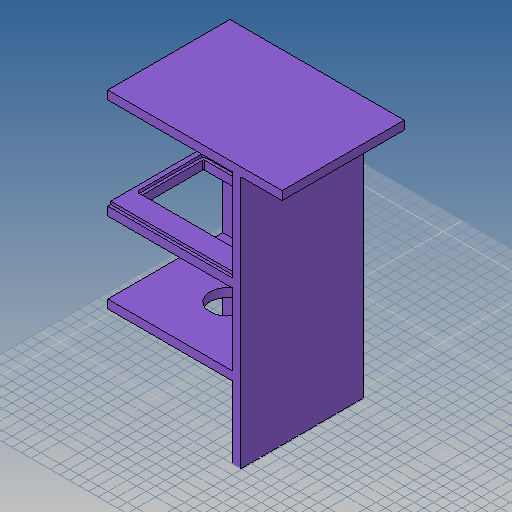
# Autodesk Inventor part: Korpus_Einbau
Saved by Autodesk Inventor 2019 (Build 230136000, 136)
## iProperties
Created: 2020-08-02
Part Number: Korpus_Einbau
Material: Generisch
Document SubType Name: Modeling
Designer: Stefan
Density: 1 g/cm^3
Appearance: Violett
Mass: 7933.41 g
Surface Area: 9734.6 cm^2
Volume: 7933.41 cm^3
Author: Stefan
Autodesk Inventor part; units mm, degrees
ref_plane "YZ Plane" through (0, 0, 0) normal (1, 0, 0) x (0, 1, 0)
ref_plane "XZ Plane" through (0, 0, 0) normal (0, 1, 0) x (-1, 0, 0)
ref_plane "XY Plane" through (0, 0, 0) normal (0, 0, 1) x (1, 0, 0)
sketch "Skizze1" plane through (0, 0, 0) normal (1, 0, 0) x (0, 1, 0)
  line L0 (0, 0) -> (18, 0)
  line L1 (18, 0) -> (18, 240)
  line L2 (18, 240) -> (0, 240)
  line L3 (0, 240) -> (0, 0)
  line L4 (378, 0) -> (-150, 0)
  line L5 (-150, -15) -> (378, -15)
  line L6 (378, -15) -> (378, 0)
  line L7 (378, -15) -> (378, 240)
  line L8 (378, 240) -> (396, 240)
  line L9 (396, 240) -> (396, -15)
  line L10 (396, -15) -> (378, -15)
  line L11 (-150, 0) -> (-150, -15)
  line L12 (186, 0) -> (168, 0)
  line L13 (168, 0) -> (168, 240)
  line L14 (168, 240) -> (186, 240)
  line L15 (186, 240) -> (186, 0)
  dimension "d0" = 18
  dimension "d1" = 15
  dimension "d2" = 18
  dimension "d5" = 255
  dimension "d6" = 360
  dimension "d23" = 150
  dimension "d49" = 18
  dimension "d50" = 150
  dimension "d51" = 192
  dimension "d52" = 255
  constraints: 32 end point, 6 parallel, 4 horizontal, 3 collinear, 2 perpendicular, 2 point on line, 1 vertical
  measures "d0" distance between parallel lines of L3 L1
  measures "d1" distance of L5.end L4.start
  measures "d2" distance of L7.end L8.end
  measures "d5" distance between parallel lines of L5 L2
  measures "d6" distance between parallel lines of L1 L7
  measures "d23" distance between parallel lines of L11 L3
  measures "d49" distance between parallel lines of L13 L15
  measures "d50" distance between parallel lines of L1 L13
  measures "d51" distance between parallel lines of L15 L7
  measures "d52" distance between parallel lines of L14 L5
extrude "Extrusion1" add sketch "Skizze1" against normal blind 260
extrude "Extrusion7" add sketch "Skizze1" along normal blind 104 contours L6 L7 L8 L9 L10
sketch "Skizze2" plane through (0, 0, 0) normal (0, -1, 0) x (1, 0, 0)
  line L0 (0, 0) -> (-260, 0) projected
  line L1 (0, 240) -> (-260, 240) projected
  circle A0 centre (-130, 120) radius 36.5
  line L2 (-130, 240) -> (-130, 0) construction
  point P0 (240, 0)
  dimension "d9" = 73
  constraints: 3 midpoint, 2 end point, 1 centre point, 1 coincident
  measures "d9" diameter of A0
extrude "Extrusion2" cut sketch "Skizze2" against normal up to surface (18 mm away)
sketch "Skizze4" plane through (0, 18, 0) normal (0, 0, 1) x (1, 0, 0)
  circle A0 centre (-140.0937, 257.9889) radius 25
  ellipse E0 centre (-140.0937, 257.9889) end of major axis (-140.0937, 283.4889) minor radius 25.5 projected
  dimension "d16" = 50
  constraints: 1 centre point, 1 coincident, 1 other
  measures "d16" diameter of A0
extrude "Extrusion4" cut sketch "Skizze4" against normal up to surface (15 mm away) contours A0
sketch "Skizze6" plane through (0, 0, 0) normal (1, 0, 0) x (0, 0, -1)
  line L0 (15, -150) -> (15, 378) projected
  line L1 (-240, 378) -> (15, 378)
  line L2 (15, 378) -> (15, -150)
  line L3 (15, -150) -> (-240, -150)
  line L4 (-240, -150) -> (-240, 378)
  line L5 (15, 396) -> (15, 378) projected
  line L6 (15, 378) -> (15, -150) projected
  line L7 (15, -150) -> (0, -150) projected
  line L8 (0, 0) -> (-240, 0) projected
  line L9 (-240, 0) -> (-240, 18) projected
  line L10 (-240, 18) -> (0, 18) projected
  line L11 (0, 186) -> (0, 378) projected
  line L12 (0, 378) -> (-240, 378) projected
  line L13 (-240, 378) -> (-240, 396) projected
  line L14 (-240, 396) -> (15, 396) projected
  line L15 (15, 378) -> (0, 378) projected
  line L16 (-240, 168) -> (-240, 186) projected
  line L17 (-240, 186) -> (0, 186) projected
  line L18 (0, 18) -> (0, 168) projected
  line L19 (0, 168) -> (-240, 168) projected
  line L20 (0, -150) -> (0, 0) projected
  constraints: 8 end point, 2 parallel, 1 collinear, 1 horizontal, 1 perpendicular
extrude "Extrusion8" add sketch "Skizze6" along normal blind 18
sketch "Skizze9" plane through (-260, 186, 240) normal (0, 1, 0) x (1, 0, 0)
  line L0 (260, 240) -> (0, 240) projected
  line L1 (260, 0) -> (0, 0) projected
  line L2 (250, 185) -> (250, 55)
  line L3 (245, 50) -> (15, 50)
  line L4 (10, 55) -> (10, 185)
  line L5 (15, 190) -> (245, 190)
  line L6 (250, 190) -> (10, 50) construction
  line L7 (250, 50) -> (10, 190) construction
  arc A0 (250, 185) -> (245, 190) centre (245, 185) ccw
  arc A1 (15, 190) -> (10, 185) centre (15, 185) ccw
  arc A2 (10, 55) -> (15, 50) centre (15, 55) ccw
  arc A3 (245, 50) -> (250, 55) centre (245, 55) ccw
  line L8 (14, 184) -> (14, 56)
  line L9 (16, 54) -> (244, 54)
  line L10 (246, 56) -> (246, 184)
  line L11 (244, 186) -> (16, 186)
  line L12 (14, 186) -> (246, 54) construction
  line L13 (14, 54) -> (246, 186) construction
  arc A4 (244, 54) -> (246, 56) centre (244, 56) ccw
  arc A5 (14, 56) -> (16, 54) centre (16, 56) ccw
  arc A6 (16, 186) -> (14, 184) centre (16, 184) ccw
  arc A7 (246, 184) -> (244, 186) centre (244, 184) ccw
  line L14 (244, 182) -> (244, 58)
  line L15 (242, 56) -> (18, 56)
  line L16 (16, 58) -> (16, 182)
  line L17 (18, 184) -> (242, 184)
  line L18 (244, 184) -> (16, 56) construction
  line L19 (244, 56) -> (16, 184) construction
  arc A8 (242, 56) -> (244, 58) centre (242, 58) ccw
  arc A9 (16, 58) -> (18, 56) centre (18, 58) ccw
  arc A10 (18, 184) -> (16, 182) centre (18, 182) ccw
  arc A11 (244, 182) -> (242, 184) centre (242, 182) ccw
  line L20 (130, 0) -> (130, 240) construction
  line L21 (0, 240) -> (260, 240)
  line L22 (260, 240) -> (260, 0)
  line L23 (260, 0) -> (0, 0)
  line L24 (0, 0) -> (0, 240)
  line L25 (260, 240) -> (260, 0) projected
  line L26 (0, 0) -> (260, 0)
  line L27 (260, 0) -> (260, 6)
  line L28 (260, 6) -> (0, 6)
  line L29 (0, 6) -> (0, 0)
  point P0 (130, 120)
  dimension "d53" = 140
  dimension "d54" = 240
  dimension "d55" = 5
  dimension "d56" = 232
  dimension "d57" = 132
  dimension "d58" = 2
  dimension "d59" = 128
  dimension "d60" = 228
  dimension "d61" = 2
  dimension "d67" = 6
  constraints: 54 end point, 25 point on line, 24 point on circle, 24 tangent, 12 centre point, 12 parallel, 9 equal radius, 9 midpoint, 5 perpendicular, 3 horizontal
  measures "d53" distance of L6.end L7.end
  measures "d54" distance of L7.start L6.end
  measures "d55" radius of A0
  measures "d56" distance of L13.start L12.end
  measures "d57" distance of L12.end L13.end
  measures "d58" radius of A4
  measures "d59" distance of L18.end L19.end
  measures "d60" distance of L19.start L18.end
  measures "d61" radius of A8
  measures "d67" distance between parallel lines of L1 L28
extrude "Extrusion11" cut sketch "Skizze9" against normal up to surface (18 mm away) contours L14 A8 L15 A9 L16 A10 L17 A11
extrude "Extrusion12" add sketch "Skizze9" along normal blind 6 contours L22 L28 L24 L0
equation "\"d0\" = case_thickness"
equation "\"d1\" = inner_thickness"
equation "\"d2\" = case_thickness"
equation "\"d5\" = inner_depth"
equation "\"d49\" = case_thickness"
equation "\"d52\" = inner_depth"
equation "\"d7\" = inner_width"
equation "\"d26\" = -2 * case_thickness + case_width - inner_width"
equation "\"d10\" = case_width - 2 * case_thickness"
equation "\"d16\" = ht_diameter"
equation "\"d17\" = case_width - 2 * case_thickness"
equation "\"d28\" = case_thickness"
equation "\"d67\" = mdf_thickness"
equation "\"d65\" = mdf_thickness"
equation "\"kg_thickness\" = 4.9"
equation "\"ht_diameter\" = 50"
equation "\"ht_thickness\" = 1.9"
equation "\"case_thickness\" = 18"
equation "\"inner_thickness\" = 15"
equation "\"gap_fit\" = 0.1"
equation "\"gap_slide\" = 0.2"
equation "\"gap_air\" = 1"
equation "\"bore_diameter\" = 73"
equation "\"mdf_thickness\" = 6"
equation "\"tape_width\" = 15"
equation "\"tape_thickness\" = 3"
equation "\"inner_depth\" = 255"
equation "\"inner_width\" = 260"
equation "\"case_width\" = 400"
